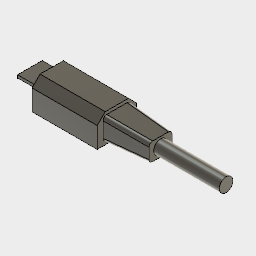
592 microUSB B Connector Cable (Autodesk Fusion 360 design; units mm, degrees)
Autodesk Fusion 360 part; units mm, degrees
sketch "Sketch1" plane through (0, 0, 0) normal (0, 0, 1) x (1, 0, 0)
  line L0 (0, 0) -> (17.9, 0)
  line L1 (17.9, 0) -> (17.9, 10.8)
  line L2 (17.9, 10.8) -> (0, 10.8)
  line L3 (0, 10.8) -> (0, 0)
  dimension "d1" = 17.9
  dimension "d2" = 10.8
  measures "d1" distance of L0.start L0.end
  measures "d2" distance of L0.start L2.end
extrude "Extrude1" add sketch "Sketch1" along normal blind 7.9
chamfer "Chamfer1" distance 2.2 angle 45 2 edges at (8.95, 10.8, 7.9) (8.95, 0, 7.9)
sketch "Sketch2" plane through (0, 0, 0) normal (-1, 0, 0) x (0, -1, 0)
  line L0 (0, 5.7) -> (-2.2, 7.9)
  line L1 (-2.2, 7.9) -> (-8.6, 7.9)
  line L2 (-8.6, 7.9) -> (-10.8, 5.7)
  line L3 (-10.8, 5.7) -> (-10.8, 0)
  line L4 (-10.8, 0) -> (0, 0)
  line L5 (0, 0) -> (0, 5.7)
  line L6 (-5.4, 7.9) -> (-5.4, 0) construction
  line L7 (-5.4, 3.95) -> (0, 3.95) construction
  line L8 (-2, 3.05) -> (-8.8, 3.05)
  line L9 (-8.8, 3.05) -> (-8.8, 4.85)
  line L10 (-8.8, 4.85) -> (-2, 4.85)
  line L11 (-2, 4.85) -> (-2, 3.05)
  line L12 (-2, 3.05) -> (-8.8, 4.85) construction
  line L13 (-8.8, 3.05) -> (-2, 4.85) construction
  point P0 (-5.4, 3.95)
  dimension "d6" = 6.8
  dimension "d7" = 1.8
  measures "d6" distance of L9.end L10.end
  measures "d7" distance of L8.end L9.end
extrude "Extrude2" add sketch "Sketch2" along normal blind 6 contours L8 L9 L10 L11
chamfer "Chamfer2" distance 1 angle 45 2 edges at (-3, 8.8, 3.05) (-3, 2, 3.05)
sketch "Sketch3" plane through (17.9, 0, 0) normal (1, 0, 0) x (0, 1, 0)
  line L0 (2.2, 7.9) -> (0, 5.7)
  line L1 (0, 5.7) -> (0, 0)
  line L2 (0, 0) -> (10.8, 0)
  line L3 (10.8, 0) -> (10.8, 5.7)
  line L4 (10.8, 5.7) -> (8.6, 7.9)
  line L5 (8.6, 7.9) -> (2.2, 7.9)
  line L6 (5.4, 7.9) -> (5.4, 0) construction
  line L7 (5.4, 3.95) -> (10.8, 3.95) construction
  line L8 (9.2, 0.85) -> (1.6, 0.85)
  line L9 (1.6, 0.85) -> (1.6, 7.05)
  line L10 (1.6, 7.05) -> (9.2, 7.05)
  line L11 (9.2, 7.05) -> (9.2, 0.85)
  line L12 (9.2, 0.85) -> (1.6, 7.05) construction
  line L13 (1.6, 0.85) -> (9.2, 7.05) construction
  point P0 (5.4, 3.95)
  dimension "d11" = 6.2
  dimension "d12" = 7.6
  measures "d11" distance of L8.end L9.end
  measures "d12" distance of L9.end L10.end
extrude "Extrude3" add sketch "Sketch3" along normal blind 12 draft -3 contours L8 L9 L10 L11
sketch "Sketch4" plane through (29.9, 0, 0) normal (1, 0, 0) x (0, 1, 0)
  line L0 (8.5711, 1.4789) -> (8.5711, 6.4211)
  line L1 (8.5711, 6.4211) -> (2.2289, 6.4211)
  line L2 (2.2289, 6.4211) -> (2.2289, 1.4789)
  line L3 (2.2289, 1.4789) -> (8.5711, 1.4789)
  line L4 (5.4, 6.4211) -> (5.4, 1.4789) construction
  line L5 (2.2289, 3.95) -> (8.5711, 3.95) construction
  circle A0 centre (5.4, 3.95) radius 1.9
  dimension "d15" = 3.8
  measures "d15" diameter of A0
extrude "Extrude4" add sketch "Sketch4" along normal blind 18 contours A0
fillet "Fillet1" radius 1 4 edges at (23.9, 1.9144, 6.7356) (23.9, 8.8856, 6.7356) (23.9, 1.9144, 1.1644) (23.9, 8.8856, 1.1644)
